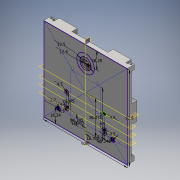
# Autodesk Inventor part: Complete Lifting Chassis with Balance and Variability
Saved by Autodesk Inventor 2016 (Build 200138000, 138)
## iProperties
Created: 2016-03-31
Part Number: Complete Lifting Chassis with Balance and Variability
Material: Generic
Document SubType Name: Modeling
Designer: Kenneth Daniel
Density: 1 g/cm^3
Appearance: Default
Author: Kenneth Daniel
## iProperties of the stored document Complete Lifting Chassis with Balance and Variability_3DPrint.ipt
Created: 2016-03-31
Part Number: Complete Lifting Chassis with Balance and Variability_3DPrint
Material: Generic
Document SubType Name: Modeling
Designer: Kenneth Daniel
Density: 1 g/cm^3
Appearance: Default
Author: Kenneth Daniel
Autodesk Inventor part; units mm, degrees
(part 1 of 2)
ref_plane "YZ Plane" through (0, 0, 0) normal (1, 0, 0) x (0, 1, 0)
ref_plane "XZ Plane" through (0, 0, 0) normal (0, 1, 0) x (-1, 0, 0)
sketch "Sketch1" plane through (0, 0, 0) normal (0, 1, 0) x (-1, 0, 0)
  line L0 (-46.4, 46.4) -> (-46.4, -46.4)
  line L1 (-46.4, -46.4) -> (46.4, -46.4)
  line L2 (46.4, -46.4) -> (46.4, 46.4)
  line L3 (46.4, 46.4) -> (-46.4, 46.4)
  line L4 (-46.4, 46.4) -> (46.4, -46.4) construction
  line L5 (-46.4, -46.4) -> (46.4, 46.4) construction
  line L6 (46.4, -46.4) -> (46.4, -30.16) construction
  line L7 (46.4, -30.16) -> (-46.4, -30.16) construction
  circle A0 centre (30.16, -30.16) radius 1.6
  circle A1 centre (30.16, -30.16) radius 2.2
  circle A2 centre (-30.16, -30.16) radius 1.6
  circle A3 centre (-30.16, -30.16) radius 2.2
  line L8 (0, 0) -> (0, -36.813) construction
  line L9 (0, -36.813) -> (16.702, -36.813) construction
  line L10 (0, -36.813) -> (-16.702, -36.813) construction
  line L11 (-16.702, -36.813) -> (-16.702, 14.187) construction
  line L12 (16.702, -36.813) -> (16.702, 14.187) construction
  line L13 (16.702, 14.187) -> (-16.702, 14.187) construction
  line L14 (16.702, -36.813) -> (16.702, -25.568) construction
  line L15 (16.702, -25.568) -> (21.202, -25.568) construction
  circle A4 centre (21.202, -25.568) radius 2.25
  line L16 (-16.702, -36.813) -> (-16.702, -25.568) construction
  line L17 (-16.702, -25.568) -> (-21.202, -25.568) construction
  line L18 (21.202, -25.568) -> (21.202, -9.693) construction
  circle A5 centre (21.202, -9.693) radius 2.25
  line L19 (-21.202, -25.568) -> (-21.202, -9.693) construction
  circle A6 centre (-21.202, -9.693) radius 2.25
  circle A7 centre (-21.202, -25.568) radius 2.25
  line L20 (0, 46.4) -> (0, 28.15) construction
  circle A8 centre (0, 28.15) radius 9.75
  circle A9 centre (0, 28.15) radius 6.2
  dimension "d0" = 92.8
  dimension "d1" = 92.8
  dimension "d2" = 16.24
  dimension "d3" = 3.2
  dimension "d4" = 4.4
  dimension "d5" = 3.2
  dimension "d6" = 4.4
  dimension "d7" = 36.813
  dimension "d8" = 16.702
  dimension "d9" = 16.702
  dimension "d10" = 51
  dimension "d11" = 11.245
  dimension "d12" = 4.5
  dimension "d13" = 4.5
  dimension "d15" = 4.5
  dimension "d16" = 11.245
  dimension "d18" = 15.875
  dimension "d19" = 4.5
  dimension "d22" = 4.5
  dimension "d23" = 4.5
  dimension "d24" = 18.25
  dimension "d25" = 19.5
  dimension "d26" = 12.4
  constraints: 42 end point, 10 centre point, 8 coincident, 8 point on line, 7 vertical, 5 perpendicular, 3 midpoint, 2 horizontal, 2 parallel
  measures "d0" distance of L0.start L0.end
  measures "d1" distance of L1.end L0.end
  measures "d2" distance of L1.end L6.end
  measures "d3" diameter of A0
  measures "d4" diameter of A1
  measures "d5" diameter of A2
  measures "d6" diameter of A3
  measures "d7" distance of L8.start L8.end
  measures "d8" distance of L8.end L9.end
  measures "d9" distance of L8.end L10.end
  measures "d10" distance of L10.end L11.end
  measures "d11" distance of L9.end L14.end
  measures "d12" distance of L14.end L15.end
  measures "d13" diameter of A4
  measures "d15" distance of L16.end L17.end
  measures "d16" distance of L10.end L16.end
  measures "d18" distance of L18.start L18.end
  measures "d19" diameter of A5
  measures "d22" diameter of A6
  measures "d23" diameter of A7
  measures "d24" distance of L20.start L20.end
  measures "d25" diameter of A8
  measures "d26" diameter of A9
extrude "Extrusion1" add sketch "Sketch1" along normal blind 5 contours L3 L2 L1 L0
extrude "Extrusion2" add sketch "Sketch1" along normal blind 1 contours A8
sketch "Sketch2" plane through (0, 1, 28.15) normal (0, 1, 0) x (1, 0, 0)
  circle A0 centre (0, 0) radius 9.75 projected
  circle A1 centre (0, 0) radius 6.2 projected
  circle A2 centre (0, 0) radius 6.2 projected
  circle A3 centre (0, 0) radius 9.75 projected
  line L0 (16.0737, 0.15) -> (6.1982, 0.15)
  line L1 (5.3373, 0.15) -> (5.3373, -0.15)
  line L2 (6.1982, -0.15) -> (16.0737, -0.15)
  line L3 (16.0737, -0.15) -> (16.0737, 0.15)
  line L4 (16.0737, 0.15) -> (5.3373, -0.15) construction
  line L5 (5.3373, 0.15) -> (16.0737, -0.15) construction
  circle A4 centre (0, 0) radius 6.2
  circle A5 centre (0, 0) radius 9.75
  circle A6 centre (0, 0) radius 6.2 projected
  line L6 (5.3373, 0.15) -> (9.7488, 0.15)
  line L7 (5.3373, -0.15) -> (9.7488, -0.15)
  arc A7 (4, -0.15) -> (3.9887, 0.15) centre (0, -0.15) ccw
  line L8 (5.3373, -0.15) -> (4, -0.15)
  line L9 (5.3373, 0.15) -> (3.9887, 0.15)
  point P0 (0, 28.15)
  point P1 (10.7055, 0)
  dimension "d35" = 0.3
  dimension "d43" = 8
  constraints: 20 end point, 8 point on circle, 3 centre point, 3 parallel, 3 point on line, 2 coincident, 2 midpoint, 1 horizontal, 1 perpendicular
  measures "d35" distance of L1.end L1.start
  measures "d43" diameter of A7
extrude "Extrusion5" add sketch "Sketch2" along normal up to surface (4 mm away) contours A0 L2 A1 L0 | A1 L7 L1 L6 | L1 L8 A7 L9 picked at (7.3832, -0.0333)
pattern_circular "Circular Pattern2" count 30 over 360 about axis through (0, 0, 28.15) along (0, 1, 0) of "Extrusion5"
sketch "Sketch4" plane through (0, 0, 0) normal (0, -1, 0) x (1, 0, 0)
  circle A0 centre (0, 28.15) radius 6.2 projected
  circle A1 centre (21.202, -25.568) radius 2.25 projected
  circle A2 centre (21.202, -9.693) radius 2.25 projected
  circle A3 centre (-21.202, -9.693) radius 2.25 projected
  circle A4 centre (-21.202, -25.568) radius 2.25 projected
  circle A5 centre (30.16, -30.16) radius 2.2 projected
  circle A6 centre (-30.16, -30.16) radius 2.2 projected
  line L0 (46.4, 46.4) -> (46.4, -46.4) projected
  line L1 (-46.4, 46.4) -> (46.4, 46.4) projected
  line L2 (-46.4, -46.4) -> (-46.4, 46.4) projected
  line L3 (46.4, -46.4) -> (-46.4, -46.4) projected
  circle A7 centre (0, 28.15) radius 3.9916
  circle A8 centre (0, 28.15) radius 4.3916
  point P0 (0, 0)
  dimension "d49" = 0.4
  constraints: 2 centre point, 1 coincident
  measures "d49" radial gap between concentric circles of A7 A8
extrude "Extrusion6" add sketch "Sketch4" against normal up to surface (1 mm away) contours A8
sketch "Sketch5" plane through (0, 5, 0) normal (0, 1, 0) x (1, 0, 0)
  circle A0 centre (0, -28.1477) radius 9.8088
  circle A1 centre (0, -28.1477) radius 6.2001
  point P0 (0, 0)
  constraints: 2 centre point, 1 coincident
extrude "Extrusion7" add sketch "Sketch5" against normal blind 0.5
sketch "Sketch6" plane through (0, 5, 0) normal (0, 1, 0) x (1, 0, 0)
  line L0 (46.4, -46.4) -> (46.4, 46.4) projected
  line L1 (46.4, 46.4) -> (-46.4, 46.4) projected
  line L2 (-46.4, 46.4) -> (-46.4, -46.4) projected
  line L3 (-46.4, -46.4) -> (46.4, -46.4) projected
  circle A0 centre (-30.16, 30.16) radius 2.2 projected
  circle A1 centre (30.16, 30.16) radius 2.2 projected
  circle A2 centre (-21.202, 25.568) radius 2.25 projected
  circle A3 centre (-21.202, 9.693) radius 2.25 projected
  circle A4 centre (21.202, 9.693) radius 2.25 projected
  circle A5 centre (21.202, 25.568) radius 2.25 projected
  line L4 (-3.9887, -28.3) -> (-6.1982, -28.3) projected
  arc A6 (-4, -28) -> (-3.9887, -28.3) centre (0, -28) ccw projected
  line L5 (-6.1983, -28) -> (-4, -28) projected
  arc A7 (-6.0944, -27.0079) -> (-6.1983, -28) centre (0, -28.1477) ccw projected
  line L6 (-3.9328, -27.4674) -> (-6.0944, -27.0079) projected
  arc A8 (-3.8814, -27.1716) -> (-3.9328, -27.4674) centre (0.0312, -28.0033) ccw projected
  line L7 (-6.0321, -26.7145) -> (-3.8814, -27.1716) projected
  arc A9 (-5.7242, -25.7656) -> (-6.0321, -26.7145) centre (0, -28.1477) ccw projected
  line L8 (-3.7049, -26.6647) -> (-5.7242, -25.7656) projected
  arc A10 (-3.5932, -26.386) -> (-3.7049, -26.6647) centre (0.061, -28.013) ccw projected
  line L9 (-5.6023, -25.4915) -> (-3.5932, -26.386) projected
  arc A11 (-5.1037, -24.6273) -> (-5.6023, -25.4915) centre (0, -28.1477) ccw projected
  line L10 (-3.3151, -25.9268) -> (-5.1037, -24.6273) projected
  arc A12 (-3.1479, -25.6775) -> (-3.3151, -25.9268) centre (0.0882, -28.0286) ccw projected
  line L11 (-4.9275, -24.3846) -> (-3.1479, -25.6775) projected
  arc A13 (-4.26, -23.6429) -> (-4.9275, -24.3846) centre (0, -28.1477) ccw projected
  line L12 (-2.7805, -25.2862) -> (-4.26, -23.6429) projected
  arc A14 (-2.5651, -25.0771) -> (-2.7805, -25.2862) centre (0.1115, -28.0496) ccw projected
  line L13 (-4.0371, -23.4421) -> (-2.5651, -25.0771) projected
  arc A15 (-3.23, -22.8555) -> (-4.0371, -23.4421) centre (0, -28.1477) ccw projected
  line L14 (-2.1243, -24.7707) -> (-3.23, -22.8555) projected
  arc A16 (-1.8701, -24.6109) -> (-2.1243, -24.7707) centre (0.1299, -28.075) ccw projected
  line L15 (-2.9702, -22.7054) -> (-1.8701, -24.6109) projected
  arc A17 (-2.0587, -22.2994) -> (-2.9702, -22.7054) centre (0, -28.1477) ccw projected
  line L16 (-1.3752, -24.4028) -> (-2.0587, -22.2994) projected
  arc A18 (-1.0934, -24.2994) -> (-1.3752, -24.4028) centre (0.1427, -28.1036) ccw projected
  line L17 (-1.7734, -22.2067) -> (-1.0934, -24.2994) projected
  arc A19 (-0.7973, -21.9991) -> (-1.7734, -22.2067) centre (0, -28.1477) ccw projected
  line L18 (-0.5661, -24.1988) -> (-0.7973, -21.9991) projected
  arc A20 (-0.2689, -24.1562) -> (-0.5661, -24.1988) centre (0.1492, -28.1343) ccw projected
  line L19 (-0.499, -21.9677) -> (-0.2689, -24.1562) projected
  arc A21 (0.499, -21.9677) -> (-0.499, -21.9677) centre (0, -28.1477) ccw projected
  line L20 (0.2678, -24.1674) -> (0.499, -21.9677) projected
  arc A22 (0.5673, -24.1876) -> (0.2678, -24.1674) centre (0.1492, -28.1657) ccw projected
  line L21 (0.7973, -21.9991) -> (0.5673, -24.1876) projected
  arc A23 (1.7734, -22.2067) -> (0.7973, -21.9991) centre (0, -28.1477) ccw projected
  line L22 (1.0899, -24.3101) -> (1.7734, -22.2067) projected
  arc A24 (1.3787, -24.3921) -> (1.0899, -24.3101) centre (0.1427, -28.1964) ccw projected
  line L23 (2.0587, -22.2994) -> (1.3787, -24.3921) projected
  arc A25 (2.9702, -22.7054) -> (2.0587, -22.2994) centre (0, -28.1477) ccw projected
  line L24 (1.8645, -24.6207) -> (2.9702, -22.7054) projected
  arc A26 (2.1299, -24.7609) -> (1.8645, -24.6207) centre (0.1299, -28.225) ccw projected
  line L25 (3.23, -22.8555) -> (2.1299, -24.7609) projected
  arc A27 (4.0371, -23.4421) -> (3.23, -22.8555) centre (0, -28.1477) ccw projected
  line L26 (2.5575, -25.0854) -> (4.0371, -23.4421) projected
  arc A28 (2.788, -25.2778) -> (2.5575, -25.0854) centre (0.1115, -28.2504) ccw projected
  line L27 (4.26, -23.6429) -> (2.788, -25.2778) projected
  arc A29 (4.9275, -24.3846) -> (4.26, -23.6429) centre (0, -28.1477) ccw projected
  line L28 (3.1388, -25.6841) -> (4.9275, -24.3846) projected
  arc A30 (3.3242, -25.9202) -> (3.1388, -25.6841) centre (0.0882, -28.2714) ccw projected
  line L29 (5.1037, -24.6273) -> (3.3242, -25.9202) projected
  arc A31 (5.6023, -25.4915) -> (5.1037, -24.6273) centre (0, -28.1477) ccw projected
  line L30 (3.5829, -26.3906) -> (5.6023, -25.4915) projected
  arc A32 (3.7152, -26.6601) -> (3.5829, -26.3906) centre (0.061, -28.287) ccw projected
  line L31 (5.7242, -25.7656) -> (3.7152, -26.6601) projected
  arc A33 (6.0321, -26.7145) -> (5.7242, -25.7656) centre (0, -28.1477) ccw projected
  line L32 (3.8704, -27.174) -> (6.0321, -26.7145) projected
  arc A34 (3.9438, -27.4651) -> (3.8704, -27.174) centre (0.0312, -28.2967) ccw projected
  line L33 (6.0944, -27.0079) -> (3.9438, -27.4651) projected
  arc A35 (6.1983, -28) -> (6.0944, -27.0079) centre (0, -28.1477) ccw projected
  line L34 (3.9887, -28) -> (6.1983, -28) projected
  arc A36 (4, -28.3) -> (3.9887, -28) centre (0, -28.3) ccw projected
  line L35 (6.1982, -28.3) -> (4, -28.3) projected
  arc A37 (6.0936, -29.2919) -> (6.1982, -28.3) centre (0, -28.1477) ccw projected
  line L36 (3.9328, -28.8326) -> (6.0936, -29.2919) projected
  arc A38 (3.8814, -29.1284) -> (3.9328, -28.8326) centre (-0.0312, -28.2967) ccw projected
  line L37 (6.0311, -29.5853) -> (3.8814, -29.1284) projected
  arc A39 (5.7226, -30.5337) -> (6.0311, -29.5853) centre (0, -28.1477) ccw projected
  line L38 (3.7049, -29.6353) -> (5.7226, -30.5337) projected
  arc A40 (3.5932, -29.914) -> (3.7049, -29.6353) centre (-0.061, -28.287) ccw projected
  line L39 (5.6005, -30.8077) -> (3.5932, -29.914) projected
  arc A41 (5.1016, -31.6711) -> (5.6005, -30.8077) centre (0, -28.1477) ccw projected
  line L40 (3.3151, -30.3732) -> (5.1016, -31.6711) projected
  arc A42 (3.1479, -30.6225) -> (3.3151, -30.3732) centre (-0.0882, -28.2714) ccw projected
  line L41 (4.9252, -31.9138) -> (3.1479, -30.6225) projected
  arc A43 (4.2578, -32.6546) -> (4.9252, -31.9138) centre (0, -28.1477) ccw projected
  line L42 (2.7805, -31.0138) -> (4.2578, -32.6546) projected
  arc A44 (2.5651, -31.2229) -> (2.7805, -31.0138) centre (-0.1115, -28.2504) ccw projected
  line L43 (4.0348, -32.8553) -> (2.5651, -31.2229) projected
  arc A45 (3.228, -33.4411) -> (4.0348, -32.8553) centre (0, -28.1477) ccw projected
  line L44 (2.1243, -31.5293) -> (3.228, -33.4411) projected
  arc A46 (1.8701, -31.6891) -> (2.1243, -31.5293) centre (-0.1299, -28.225) ccw projected
  line L45 (2.9682, -33.5911) -> (1.8701, -31.6891) projected
  arc A47 (2.0573, -33.9964) -> (2.9682, -33.5911) centre (0, -28.1477) ccw projected
  line L46 (1.3752, -31.8972) -> (2.0573, -33.9964) projected
  arc A48 (1.0934, -32.0006) -> (1.3752, -31.8972) centre (-0.1427, -28.1964) ccw projected
  line L47 (1.772, -34.0891) -> (1.0934, -32.0006) projected
  arc A49 (0.7968, -34.2963) -> (1.772, -34.0891) centre (0, -28.1477) ccw projected
  line L48 (0.5661, -32.1012) -> (0.7968, -34.2963) projected
  arc A50 (0.2689, -32.1438) -> (0.5661, -32.1012) centre (-0.1492, -28.1657) ccw projected
  line L49 (0.4985, -34.3277) -> (0.2689, -32.1438) projected
  arc A51 (-0.4985, -34.3277) -> (0.4985, -34.3277) centre (0, -28.1477) ccw projected
  line L50 (-0.2678, -32.1326) -> (-0.4985, -34.3277) projected
  arc A52 (-0.5673, -32.1124) -> (-0.2678, -32.1326) centre (-0.1492, -28.1343) ccw projected
  line L51 (-0.7968, -34.2963) -> (-0.5673, -32.1124) projected
  arc A53 (-1.772, -34.0891) -> (-0.7968, -34.2963) centre (0, -28.1477) ccw projected
  line L52 (-1.0899, -31.9899) -> (-1.772, -34.0891) projected
  arc A54 (-1.3787, -31.9079) -> (-1.0899, -31.9899) centre (-0.1427, -28.1036) ccw projected
  line L53 (-2.0573, -33.9964) -> (-1.3787, -31.9079) projected
  arc A55 (-2.9682, -33.5911) -> (-2.0573, -33.9964) centre (0, -28.1477) ccw projected
  line L54 (-1.8645, -31.6793) -> (-2.9682, -33.5911) projected
  arc A56 (-2.1299, -31.5391) -> (-1.8645, -31.6793) centre (-0.1299, -28.075) ccw projected
  line L55 (-3.228, -33.4411) -> (-2.1299, -31.5391) projected
  arc A57 (-4.0348, -32.8553) -> (-3.228, -33.4411) centre (0, -28.1477) ccw projected
  line L56 (-2.5575, -31.2146) -> (-4.0348, -32.8553) projected
  arc A58 (-2.788, -31.0222) -> (-2.5575, -31.2146) centre (-0.1115, -28.0496) ccw projected
  line L57 (-4.2578, -32.6546) -> (-2.788, -31.0222) projected
  arc A59 (-4.9252, -31.9138) -> (-4.2578, -32.6546) centre (0, -28.1477) ccw projected
  line L58 (-3.1388, -30.6159) -> (-4.9252, -31.9138) projected
  arc A60 (-3.3242, -30.3798) -> (-3.1388, -30.6159) centre (-0.0882, -28.0286) ccw projected
  line L59 (-5.1016, -31.6711) -> (-3.3242, -30.3798) projected
  arc A61 (-5.6005, -30.8077) -> (-5.1016, -31.6711) centre (0, -28.1477) ccw projected
  line L60 (-3.5829, -29.9094) -> (-5.6005, -30.8077) projected
  arc A62 (-3.7152, -29.6399) -> (-3.5829, -29.9094) centre (-0.061, -28.013) ccw projected
  line L61 (-5.7226, -30.5337) -> (-3.7152, -29.6399) projected
  arc A63 (-6.0311, -29.5853) -> (-5.7226, -30.5337) centre (0, -28.1477) ccw projected
  line L62 (-3.8704, -29.126) -> (-6.0311, -29.5853) projected
  arc A64 (-3.9438, -28.8349) -> (-3.8704, -29.126) centre (-0.0312, -28.0033) ccw projected
  line L63 (-6.0936, -29.2919) -> (-3.9438, -28.8349) projected
  arc A65 (-6.1982, -28.3) -> (-6.0936, -29.2919) centre (0, -28.1477) ccw projected
  circle A66 centre (-21.202, 9.693) radius 2.25 projected
  line L64 (-19.3895, 11.0261) -> (-23.0065, 8.349) construction
  line L65 (-19.332, 10.9442) -> (-20.3393, 10.1987)
  line L66 (-21.9377, 9.0157) -> (-22.945, 8.2701)
  line L67 (-19.4505, 11.1054) -> (-20.4572, 10.3603)
  line L68 (-22.0578, 9.1756) -> (-23.0644, 8.4305)
  arc A67 (-22.0578, 9.1756) -> (-21.9377, 9.0157) centre (-21.202, 9.693) ccw
  arc A68 (-20.3393, 10.1987) -> (-20.4572, 10.3603) centre (-21.202, 9.693) ccw
  point P0 (0, 0)
  constraints: 16 point on circle, 10 end point, 2 centre point, 2 parallel, 1 coincident, 1 other
extrude "Extrusion8" add sketch "Sketch6" against normal up to surface (5 mm away) contours L65 A68 L67 A3 | A3 L68 A67 L66
pattern_circular "Circular Pattern3" count 10 over 360 about axis through (-21.202, 0, -9.693) along (0, 1, 0) of "Extrusion8"
ref_plane "Work Plane3" through (-21.202, 0, -9.693) normal (0, 0, 1) x (1, 0, 0)
ref_plane "Work Plane5" through (-21.202, 0, -17.6305) normal (0, 0, 1) x (1, 0, 0)
ref_plane "Work Plane4" through (-21.202, 0, -25.568) normal (0, 0, 1) x (1, 0, 0)
mirror "Mirror1" about plane through (-21.202, 0, -17.6305) normal (0, 0, 1) of "Extrusion8", "Circular Pattern3"
ref_plane "Work Plane6" through (0, 0, -46.4) normal (-1, 0, 0) x (0, 0, 1)
mirror "Mirror2" about plane through (0, 0, -46.4) normal (-1, 0, 0) of "Extrusion8", "Circular Pattern3", "Mirror1"
sketch "Sketch7" plane through (0, 5, 0) normal (0, 1, 0) x (1, 0, 0)
  arc A0 (20.3393, 25.0623) -> (20.4663, 24.8907) centre (21.202, 25.568) ccw projected
  line L0 (20.3393, 25.0623) -> (19.332, 24.3168) projected
  arc A1 (18.9556, 25.4414) -> (19.332, 24.3168) centre (21.202, 25.568) ccw projected
  line L1 (18.9556, 25.4414) -> (20.2087, 25.4525) projected
  arc A2 (20.2068, 25.666) -> (20.2087, 25.4525) centre (21.202, 25.568) ccw projected
  line L2 (20.2068, 25.666) -> (18.9537, 25.6549) projected
  arc A3 (19.3102, 26.786) -> (18.9537, 25.6549) centre (21.202, 25.568) ccw projected
  line L3 (19.3102, 26.786) -> (20.3305, 26.0584) projected
  arc A4 (20.4545, 26.2322) -> (20.3305, 26.0584) centre (21.202, 25.568) ccw projected
  line L4 (20.4545, 26.2322) -> (19.4341, 26.9598) projected
  arc A5 (20.3874, 27.6654) -> (19.4341, 26.9598) centre (21.202, 25.568) ccw projected
  line L5 (20.3874, 27.6654) -> (20.7852, 26.477) projected
  arc A6 (20.9876, 26.5448) -> (20.7852, 26.477) centre (21.202, 25.568) ccw projected
  line L6 (20.9876, 26.5448) -> (20.5899, 27.7331) projected
  arc A7 (21.7758, 27.7436) -> (20.5899, 27.7331) centre (21.202, 25.568) ccw projected
  line L7 (21.7758, 27.7436) -> (21.3991, 26.5484) projected
  arc A8 (21.6027, 26.4842) -> (21.3991, 26.5484) centre (21.202, 25.568) ccw projected
  line L8 (21.6027, 26.4842) -> (21.9794, 27.6794) projected
  arc A9 (22.945, 26.9909) -> (21.9794, 27.6794) centre (21.202, 25.568) ccw projected
  line L9 (22.945, 26.9909) -> (21.9377, 26.2453) projected
  arc A10 (22.0647, 26.0737) -> (21.9377, 26.2453) centre (21.202, 25.568) ccw projected
  line L10 (22.0647, 26.0737) -> (23.072, 26.8192) projected
  arc A11 (23.4484, 25.6946) -> (23.072, 26.8192) centre (21.202, 25.568) ccw projected
  line L11 (23.4484, 25.6946) -> (22.1953, 25.6835) projected
  arc A12 (22.1972, 25.47) -> (22.1953, 25.6835) centre (21.202, 25.568) ccw projected
  line L12 (22.1972, 25.47) -> (23.4503, 25.4811) projected
  arc A13 (23.0938, 24.35) -> (23.4503, 25.4811) centre (21.202, 25.568) ccw projected
  line L13 (23.0938, 24.35) -> (22.0735, 25.0776) projected
  arc A14 (21.9495, 24.9038) -> (22.0735, 25.0776) centre (21.202, 25.568) ccw projected
  line L14 (21.9495, 24.9038) -> (22.9699, 24.1762) projected
  arc A15 (22.0166, 23.4706) -> (22.9699, 24.1762) centre (21.202, 25.568) ccw projected
  line L15 (22.0166, 23.4706) -> (21.6188, 24.659) projected
  arc A16 (21.4164, 24.5912) -> (21.6188, 24.659) centre (21.202, 25.568) ccw projected
  line L16 (21.4164, 24.5912) -> (21.8141, 23.4029) projected
  arc A17 (20.6282, 23.3924) -> (21.8141, 23.4029) centre (21.202, 25.568) ccw projected
  line L17 (20.6282, 23.3924) -> (21.0049, 24.5876) projected
  arc A18 (20.8013, 24.6518) -> (21.0049, 24.5876) centre (21.202, 25.568) ccw projected
  line L18 (20.8013, 24.6518) -> (20.4246, 23.4566) projected
  arc A19 (19.459, 24.1451) -> (20.4246, 23.4566) centre (21.202, 25.568) ccw projected
  line L19 (19.459, 24.1451) -> (20.4663, 24.8907) projected
  arc A20 (-20.4663, 24.8907) -> (-20.3393, 25.0623) centre (-21.202, 25.568) ccw projected
  line L20 (-19.459, 24.1451) -> (-20.4663, 24.8907) projected
  arc A21 (-20.4246, 23.4566) -> (-19.459, 24.1451) centre (-21.202, 25.568) ccw projected
  line L21 (-20.8013, 24.6518) -> (-20.4246, 23.4566) projected
  arc A22 (-21.0049, 24.5876) -> (-20.8013, 24.6518) centre (-21.202, 25.568) ccw projected
  line L22 (-20.6282, 23.3924) -> (-21.0049, 24.5876) projected
  arc A23 (-21.8141, 23.4029) -> (-20.6282, 23.3924) centre (-21.202, 25.568) ccw projected
  line L23 (-21.4164, 24.5912) -> (-21.8141, 23.4029) projected
  arc A24 (-21.6188, 24.659) -> (-21.4164, 24.5912) centre (-21.202, 25.568) ccw projected
  line L24 (-22.0166, 23.4706) -> (-21.6188, 24.659) projected
  arc A25 (-22.9699, 24.1762) -> (-22.0166, 23.4706) centre (-21.202, 25.568) ccw projected
  line L25 (-21.9495, 24.9038) -> (-22.9699, 24.1762) projected
  arc A26 (-22.0735, 25.0776) -> (-21.9495, 24.9038) centre (-21.202, 25.568) ccw projected
  line L26 (-23.0938, 24.35) -> (-22.0735, 25.0776) projected
  arc A27 (-23.4503, 25.4811) -> (-23.0938, 24.35) centre (-21.202, 25.568) ccw projected
  line L27 (-22.1972, 25.47) -> (-23.4503, 25.4811) projected
  arc A28 (-22.1953, 25.6835) -> (-22.1972, 25.47) centre (-21.202, 25.568) ccw projected
  line L28 (-23.4484, 25.6946) -> (-22.1953, 25.6835) projected
  arc A29 (-23.072, 26.8192) -> (-23.4484, 25.6946) centre (-21.202, 25.568) ccw projected
  line L29 (-22.0647, 26.0737) -> (-23.072, 26.8192) projected
  arc A30 (-21.9377, 26.2453) -> (-22.0647, 26.0737) centre (-21.202, 25.568) ccw projected
  line L30 (-22.945, 26.9909) -> (-21.9377, 26.2453) projected
  arc A31 (-21.9794, 27.6794) -> (-22.945, 26.9909) centre (-21.202, 25.568) ccw projected
  line L31 (-21.6027, 26.4842) -> (-21.9794, 27.6794) projected
  arc A32 (-21.3991, 26.5484) -> (-21.6027, 26.4842) centre (-21.202, 25.568) ccw projected
  line L32 (-21.7758, 27.7436) -> (-21.3991, 26.5484) projected
  arc A33 (-20.5899, 27.7331) -> (-21.7758, 27.7436) centre (-21.202, 25.568) ccw projected
  line L33 (-20.9876, 26.5448) -> (-20.5899, 27.7331) projected
  arc A34 (-20.7852, 26.477) -> (-20.9876, 26.5448) centre (-21.202, 25.568) ccw projected
  line L34 (-20.3874, 27.6654) -> (-20.7852, 26.477) projected
  arc A35 (-19.4341, 26.9598) -> (-20.3874, 27.6654) centre (-21.202, 25.568) ccw projected
  line L35 (-20.4545, 26.2322) -> (-19.4341, 26.9598) projected
  arc A36 (-20.3305, 26.0584) -> (-20.4545, 26.2322) centre (-21.202, 25.568) ccw projected
  line L36 (-19.3102, 26.786) -> (-20.3305, 26.0584) projected
  arc A37 (-18.9537, 25.6549) -> (-19.3102, 26.786) centre (-21.202, 25.568) ccw projected
  line L37 (-20.2068, 25.666) -> (-18.9537, 25.6549) projected
  arc A38 (-20.2087, 25.4525) -> (-20.2068, 25.666) centre (-21.202, 25.568) ccw projected
  line L38 (-18.9556, 25.4414) -> (-20.2087, 25.4525) projected
  arc A39 (-19.332, 24.3168) -> (-18.9556, 25.4414) centre (-21.202, 25.568) ccw projected
  line L39 (-20.3393, 25.0623) -> (-19.332, 24.3168) projected
  arc A40 (-20.3393, 10.1987) -> (-20.4663, 10.3703) centre (-21.202, 9.693) ccw projected
  line L40 (-20.3393, 10.1987) -> (-19.332, 10.9442) projected
  arc A41 (-18.9556, 9.8196) -> (-19.332, 10.9442) centre (-21.202, 9.693) ccw projected
  line L41 (-18.9556, 9.8196) -> (-20.2087, 9.8085) projected
  arc A42 (-20.2068, 9.595) -> (-20.2087, 9.8085) centre (-21.202, 9.693) ccw projected
  line L42 (-20.2068, 9.595) -> (-18.9537, 9.6061) projected
  arc A43 (-19.3102, 8.475) -> (-18.9537, 9.6061) centre (-21.202, 9.693) ccw projected
  line L43 (-19.3102, 8.475) -> (-20.3305, 9.2026) projected
  arc A44 (-20.4545, 9.0288) -> (-20.3305, 9.2026) centre (-21.202, 9.693) ccw projected
  line L44 (-20.4545, 9.0288) -> (-19.4341, 8.3012) projected
  arc A45 (-20.3874, 7.5956) -> (-19.4341, 8.3012) centre (-21.202, 9.693) ccw projected
  line L45 (-20.3874, 7.5956) -> (-20.7852, 8.784) projected
  arc A46 (-20.9876, 8.7162) -> (-20.7852, 8.784) centre (-21.202, 9.693) ccw projected
  line L46 (-20.9876, 8.7162) -> (-20.5899, 7.5279) projected
  arc A47 (-21.7758, 7.5174) -> (-20.5899, 7.5279) centre (-21.202, 9.693) ccw projected
  line L47 (-21.7758, 7.5174) -> (-21.3991, 8.7126) projected
  arc A48 (-21.6027, 8.7768) -> (-21.3991, 8.7126) centre (-21.202, 9.693) ccw projected
  line L48 (-21.6027, 8.7768) -> (-21.9794, 7.5816) projected
  arc A49 (-22.945, 8.2701) -> (-21.9794, 7.5816) centre (-21.202, 9.693) ccw projected
  line L49 (-22.945, 8.2701) -> (-21.9377, 9.0157) projected
  arc A50 (-22.0647, 9.1873) -> (-21.9377, 9.0157) centre (-21.202, 9.693) ccw projected
  line L50 (-22.0647, 9.1873) -> (-23.072, 8.4418) projected
  arc A51 (-23.4484, 9.5664) -> (-23.072, 8.4418) centre (-21.202, 9.693) ccw projected
  line L51 (-23.4484, 9.5664) -> (-22.1953, 9.5775) projected
  arc A52 (-22.1972, 9.791) -> (-22.1953, 9.5775) centre (-21.202, 9.693) ccw projected
  line L52 (-22.1972, 9.791) -> (-23.4503, 9.7799) projected
  arc A53 (-23.0938, 10.911) -> (-23.4503, 9.7799) centre (-21.202, 9.693) ccw projected
  line L53 (-23.0938, 10.911) -> (-22.0735, 10.1834) projected
  arc A54 (-21.9495, 10.3572) -> (-22.0735, 10.1834) centre (-21.202, 9.693) ccw projected
  line L54 (-21.9495, 10.3572) -> (-22.9699, 11.0848) projected
  arc A55 (-22.0166, 11.7904) -> (-22.9699, 11.0848) centre (-21.202, 9.693) ccw projected
  line L55 (-22.0166, 11.7904) -> (-21.6188, 10.602) projected
  arc A56 (-21.4164, 10.6698) -> (-21.6188, 10.602) centre (-21.202, 9.693) ccw projected
  line L56 (-21.4164, 10.6698) -> (-21.8141, 11.8581) projected
  arc A57 (-20.6282, 11.8686) -> (-21.8141, 11.8581) centre (-21.202, 9.693) ccw projected
  line L57 (-20.6282, 11.8686) -> (-21.0049, 10.6734) projected
  arc A58 (-20.8013, 10.6092) -> (-21.0049, 10.6734) centre (-21.202, 9.693) ccw projected
  line L58 (-20.8013, 10.6092) -> (-20.4246, 11.8044) projected
  arc A59 (-19.459, 11.1159) -> (-20.4246, 11.8044) centre (-21.202, 9.693) ccw projected
  line L59 (-19.459, 11.1159) -> (-20.4663, 10.3703) projected
  line L60 (46.4, -46.4) -> (46.4, 46.4) projected
  line L61 (46.4, 46.4) -> (-46.4, 46.4) projected
  line L62 (-46.4, 46.4) -> (-46.4, -46.4) projected
  line L63 (-46.4, -46.4) -> (46.4, -46.4) projected
  circle A60 centre (-30.16, 30.16) radius 2.2 projected
  circle A61 centre (30.16, 30.16) radius 2.2 projected
  line L64 (-3.9887, -28.3) -> (-6.1982, -28.3) projected
  arc A62 (-4, -28) -> (-3.9887, -28.3) centre (0, -28) ccw projected
  line L65 (-6.1983, -28) -> (-4, -28) projected
  arc A63 (-6.0944, -27.0079) -> (-6.1983, -28) centre (0, -28.1477) ccw projected
  line L66 (-3.9328, -27.4674) -> (-6.0944, -27.0079) projected
  arc A64 (-3.8814, -27.1716) -> (-3.9328, -27.4674) centre (0.0312, -28.0033) ccw projected
  line L67 (-6.0321, -26.7145) -> (-3.8814, -27.1716) projected
  arc A65 (-5.7242, -25.7656) -> (-6.0321, -26.7145) centre (0, -28.1477) ccw projected
  line L68 (-3.7049, -26.6647) -> (-5.7242, -25.7656) projected
  arc A66 (-3.5932, -26.386) -> (-3.7049, -26.6647) centre (0.061, -28.013) ccw projected
  line L69 (-5.6023, -25.4915) -> (-3.5932, -26.386) projected
  arc A67 (-5.1037, -24.6273) -> (-5.6023, -25.4915) centre (0, -28.1477) ccw projected
  line L70 (-3.3151, -25.9268) -> (-5.1037, -24.6273) projected
  arc A68 (-3.1479, -25.6775) -> (-3.3151, -25.9268) centre (0.0882, -28.0286) ccw projected
  line L71 (-4.9275, -24.3846) -> (-3.1479, -25.6775) projected
  arc A69 (-4.26, -23.6429) -> (-4.9275, -24.3846) centre (0, -28.1477) ccw projected
  line L72 (-2.7805, -25.2862) -> (-4.26, -23.6429) projected
  arc A70 (-2.5651, -25.0771) -> (-2.7805, -25.2862) centre (0.1115, -28.0496) ccw projected
  line L73 (-4.0371, -23.4421) -> (-2.5651, -25.0771) projected
  arc A71 (-3.23, -22.8555) -> (-4.0371, -23.4421) centre (0, -28.1477) ccw projected
  line L74 (-2.1243, -24.7707) -> (-3.23, -22.8555) projected
  arc A72 (-1.8701, -24.6109) -> (-2.1243, -24.7707) centre (0.1299, -28.075) ccw projected
  line L75 (-2.9702, -22.7054) -> (-1.8701, -24.6109) projected
  arc A73 (-2.0587, -22.2994) -> (-2.9702, -22.7054) centre (0, -28.1477) ccw projected
  line L76 (-1.3752, -24.4028) -> (-2.0587, -22.2994) projected
  arc A74 (-1.0934, -24.2994) -> (-1.3752, -24.4028) centre (0.1427, -28.1036) ccw projected
  line L77 (-1.7734, -22.2067) -> (-1.0934, -24.2994) projected
  arc A75 (-0.7973, -21.9991) -> (-1.7734, -22.2067) centre (0, -28.1477) ccw projected
  line L78 (-0.5661, -24.1988) -> (-0.7973, -21.9991) projected
  arc A76 (-0.2689, -24.1562) -> (-0.5661, -24.1988) centre (0.1492, -28.1343) ccw projected
  line L79 (-0.499, -21.9677) -> (-0.2689, -24.1562) projected
  arc A77 (0.499, -21.9677) -> (-0.499, -21.9677) centre (0, -28.1477) ccw projected
  line L80 (0.2678, -24.1674) -> (0.499, -21.9677) projected
  arc A78 (0.5673, -24.1876) -> (0.2678, -24.1674) centre (0.1492, -28.1657) ccw projected
  line L81 (0.7973, -21.9991) -> (0.5673, -24.1876) projected
  arc A79 (1.7734, -22.2067) -> (0.7973, -21.9991) centre (0, -28.1477) ccw projected
  line L82 (1.0899, -24.3101) -> (1.7734, -22.2067) projected
  arc A80 (1.3787, -24.3921) -> (1.0899, -24.3101) centre (0.1427, -28.1964) ccw projected
  line L83 (2.0587, -22.2994) -> (1.3787, -24.3921) projected
  arc A81 (2.9702, -22.7054) -> (2.0587, -22.2994) centre (0, -28.1477) ccw projected
  line L84 (1.8645, -24.6207) -> (2.9702, -22.7054) projected
  arc A82 (2.1299, -24.7609) -> (1.8645, -24.6207) centre (0.1299, -28.225) ccw projected
  line L85 (3.23, -22.8555) -> (2.1299, -24.7609) projected
  arc A83 (4.0371, -23.4421) -> (3.23, -22.8555) centre (0, -28.1477) ccw projected
  line L86 (2.5575, -25.0854) -> (4.0371, -23.4421) projected
  arc A84 (2.788, -25.2778) -> (2.5575, -25.0854) centre (0.1115, -28.2504) ccw projected
  line L87 (4.26, -23.6429) -> (2.788, -25.2778) projected
  arc A85 (4.9275, -24.3846) -> (4.26, -23.6429) centre (0, -28.1477) ccw projected
  line L88 (3.1388, -25.6841) -> (4.9275, -24.3846) projected
  arc A86 (3.3242, -25.9202) -> (3.1388, -25.6841) centre (0.0882, -28.2714) ccw projected
  line L89 (5.1037, -24.6273) -> (3.3242, -25.9202) projected
  arc A87 (5.6023, -25.4915) -> (5.1037, -24.6273) centre (0, -28.1477) ccw projected
  line L90 (3.5829, -26.3906) -> (5.6023, -25.4915) projected
  arc A88 (3.7152, -26.6601) -> (3.5829, -26.3906) centre (0.061, -28.287) ccw projected
  line L91 (5.7242, -25.7656) -> (3.7152, -26.6601) projected
  arc A89 (6.0321, -26.7145) -> (5.7242, -25.7656) centre (0, -28.1477) ccw projected
  line L92 (3.8704, -27.174) -> (6.0321, -26.7145) projected
  arc A90 (3.9438, -27.4651) -> (3.8704, -27.174) centre (0.0312, -28.2967) ccw projected
  line L93 (6.0944, -27.0079) -> (3.9438, -27.4651) projected
  arc A91 (6.1983, -28) -> (6.0944, -27.0079) centre (0, -28.1477) ccw projected
  line L94 (3.9887, -28) -> (6.1983, -28) projected
  arc A92 (4, -28.3) -> (3.9887, -28) centre (0, -28.3) ccw projected
  line L95 (6.1982, -28.3) -> (4, -28.3) projected
  arc A93 (6.0936, -29.2919) -> (6.1982, -28.3) centre (0, -28.1477) ccw projected
  line L96 (3.9328, -28.8326) -> (6.0936, -29.2919) projected
  arc A94 (3.8814, -29.1284) -> (3.9328, -28.8326) centre (-0.0312, -28.2967) ccw projected
  line L97 (6.0311, -29.5853) -> (3.8814, -29.1284) projected
  arc A95 (5.7226, -30.5337) -> (6.0311, -29.5853) centre (0, -28.1477) ccw projected
  line L98 (3.7049, -29.6353) -> (5.7226, -30.5337) projected
  arc A96 (3.5932, -29.914) -> (3.7049, -29.6353) centre (-0.061, -28.287) ccw projected
  line L99 (5.6005, -30.8077) -> (3.5932, -29.914) projected
  arc A97 (5.1016, -31.6711) -> (5.6005, -30.8077) centre (0, -28.1477) ccw projected
  line L100 (3.3151, -30.3732) -> (5.1016, -31.6711) projected
  arc A98 (3.1479, -30.6225) -> (3.3151, -30.3732) centre (-0.0882, -28.2714) ccw projected
  line L101 (4.9252, -31.9138) -> (3.1479, -30.6225) projected
  arc A99 (4.2578, -32.6546) -> (4.9252, -31.9138) centre (0, -28.1477) ccw projected
  line L102 (2.7805, -31.0138) -> (4.2578, -32.6546) projected
  arc A100 (2.5651, -31.2229) -> (2.7805, -31.0138) centre (-0.1115, -28.2504) ccw projected
  line L103 (4.0348, -32.8553) -> (2.5651, -31.2229) projected
  arc A101 (3.228, -33.4411) -> (4.0348, -32.8553) centre (0, -28.1477) ccw projected
  line L104 (2.1243, -31.5293) -> (3.228, -33.4411) projected
  arc A102 (1.8701, -31.6891) -> (2.1243, -31.5293) centre (-0.1299, -28.225) ccw projected
  line L105 (2.9682, -33.5911) -> (1.8701, -31.6891) projected
  arc A103 (2.0573, -33.9964) -> (2.9682, -33.5911) centre (0, -28.1477) ccw projected
  line L106 (1.3752, -31.8972) -> (2.0573, -33.9964) projected
  arc A104 (1.0934, -32.0006) -> (1.3752, -31.8972) centre (-0.1427, -28.1964) ccw projected
  line L107 (1.772, -34.0891) -> (1.0934, -32.0006) projected
  arc A105 (0.7968, -34.2963) -> (1.772, -34.0891) centre (0, -28.1477) ccw projected
  line L108 (0.5661, -32.1012) -> (0.7968, -34.2963) projected
  arc A106 (0.2689, -32.1438) -> (0.5661, -32.1012) centre (-0.1492, -28.1657) ccw projected
  line L109 (0.4985, -34.3277) -> (0.2689, -32.1438) projected
  arc A107 (-0.4985, -34.3277) -> (0.4985, -34.3277) centre (0, -28.1477) ccw projected
  line L110 (-0.2678, -32.1326) -> (-0.4985, -34.3277) projected
  arc A108 (-0.5673, -32.1124) -> (-0.2678, -32.1326) centre (-0.1492, -28.1343) ccw projected
  line L111 (-0.7968, -34.2963) -> (-0.5673, -32.1124) projected
  arc A109 (-1.772, -34.0891) -> (-0.7968, -34.2963) centre (0, -28.1477) ccw projected
  line L112 (-1.0899, -31.9899) -> (-1.772, -34.0891) projected
  arc A110 (-1.3787, -31.9079) -> (-1.0899, -31.9899) centre (-0.1427, -28.1036) ccw projected
  line L113 (-2.0573, -33.9964) -> (-1.3787, -31.9079) projected
  arc A111 (-2.9682, -33.5911) -> (-2.0573, -33.9964) centre (0, -28.1477) ccw projected
  line L114 (-1.8645, -31.6793) -> (-2.9682, -33.5911) projected
  arc A112 (-2.1299, -31.5391) -> (-1.8645, -31.6793) centre (-0.1299, -28.075) ccw projected
  line L115 (-3.228, -33.4411) -> (-2.1299, -31.5391) projected
  arc A113 (-4.0348, -32.8553) -> (-3.228, -33.4411) centre (0, -28.1477) ccw projected
  line L116 (-2.5575, -31.2146) -> (-4.0348, -32.8553) projected
  arc A114 (-2.788, -31.0222) -> (-2.5575, -31.2146) centre (-0.1115, -28.0496) ccw projected
  line L117 (-4.2578, -32.6546) -> (-2.788, -31.0222) projected
  arc A115 (-4.9252, -31.9138) -> (-4.2578, -32.6546) centre (0, -28.1477) ccw projected
  line L118 (-3.1388, -30.6159) -> (-4.9252, -31.9138) projected
  arc A116 (-3.3242, -30.3798) -> (-3.1388, -30.6159) centre (-0.0882, -28.0286) ccw projected
  line L119 (-5.1016, -31.6711) -> (-3.3242, -30.3798) projected
  arc A117 (-5.6005, -30.8077) -> (-5.1016, -31.6711) centre (0, -28.1477) ccw projected
  line L120 (-3.5829, -29.9094) -> (-5.6005, -30.8077) projected
  arc A118 (-3.7152, -29.6399) -> (-3.5829, -29.9094) centre (-0.061, -28.013) ccw projected
  line L121 (-5.7226, -30.5337) -> (-3.7152, -29.6399) projected
  arc A119 (-6.0311, -29.5853) -> (-5.7226, -30.5337) centre (0, -28.1477) ccw projected
  line L122 (-3.8704, -29.126) -> (-6.0311, -29.5853) projected
  arc A120 (-3.9438, -28.8349) -> (-3.8704, -29.126) centre (-0.0312, -28.0033) ccw projected
  line L123 (-6.0936, -29.2919) -> (-3.9438, -28.8349) projected
  arc A121 (-6.1982, -28.3) -> (-6.0936, -29.2919) centre (0, -28.1477) ccw projected
  arc A122 (20.4663, 10.3703) -> (20.3393, 10.1987) centre (21.202, 9.693) ccw projected
  line L124 (19.459, 11.1159) -> (20.4663, 10.3703) projected
  arc A123 (20.4246, 11.8044) -> (19.459, 11.1159) centre (21.202, 9.693) ccw projected
  line L125 (20.8013, 10.6092) -> (20.4246, 11.8044) projected
  arc A124 (21.0049, 10.6734) -> (20.8013, 10.6092) centre (21.202, 9.693) ccw projected
  line L126 (20.6282, 11.8686) -> (21.0049, 10.6734) projected
  arc A125 (21.8141, 11.8581) -> (20.6282, 11.8686) centre (21.202, 9.693) ccw projected
  line L127 (21.4164, 10.6698) -> (21.8141, 11.8581) projected
  arc A126 (21.6188, 10.602) -> (21.4164, 10.6698) centre (21.202, 9.693) ccw projected
  line L128 (22.0166, 11.7904) -> (21.6188, 10.602) projected
  arc A127 (22.9699, 11.0848) -> (22.0166, 11.7904) centre (21.202, 9.693) ccw projected
  line L129 (21.9495, 10.3572) -> (22.9699, 11.0848) projected
  arc A128 (22.0735, 10.1834) -> (21.9495, 10.3572) centre (21.202, 9.693) ccw projected
  line L130 (23.0938, 10.911) -> (22.0735, 10.1834) projected
  arc A129 (23.4503, 9.7799) -> (23.0938, 10.911) centre (21.202, 9.693) ccw projected
  line L131 (22.1972, 9.791) -> (23.4503, 9.7799) projected
  arc A130 (22.1953, 9.5775) -> (22.1972, 9.791) centre (21.202, 9.693) ccw projected
  line L132 (23.4484, 9.5664) -> (22.1953, 9.5775) projected
  arc A131 (23.072, 8.4418) -> (23.4484, 9.5664) centre (21.202, 9.693) ccw projected
  line L133 (22.0647, 9.1873) -> (23.072, 8.4418) projected
  arc A132 (21.9377, 9.0157) -> (22.0647, 9.1873) centre (21.202, 9.693) ccw projected
  line L134 (22.945, 8.2701) -> (21.9377, 9.0157) projected
  arc A133 (21.9794, 7.5816) -> (22.945, 8.2701) centre (21.202, 9.693) ccw projected
  line L135 (21.6027, 8.7768) -> (21.9794, 7.5816) projected
  arc A134 (21.3991, 8.7126) -> (21.6027, 8.7768) centre (21.202, 9.693) ccw projected
  line L136 (21.7758, 7.5174) -> (21.3991, 8.7126) projected
  arc A135 (20.5899, 7.5279) -> (21.7758, 7.5174) centre (21.202, 9.693) ccw projected
  line L137 (20.9876, 8.7162) -> (20.5899, 7.5279) projected
  arc A136 (20.7852, 8.784) -> (20.9876, 8.7162) centre (21.202, 9.693) ccw projected
  line L138 (20.3874, 7.5956) -> (20.7852, 8.784) projected
  arc A137 (19.4341, 8.3012) -> (20.3874, 7.5956) centre (21.202, 9.693) ccw projected
  line L139 (20.4545, 9.0288) -> (19.4341, 8.3012) projected
  arc A138 (20.3305, 9.2026) -> (20.4545, 9.0288) centre (21.202, 9.693) ccw projected
  line L140 (19.3102, 8.475) -> (20.3305, 9.2026) projected
  arc A139 (18.9537, 9.6061) -> (19.3102, 8.475) centre (21.202, 9.693) ccw projected
  line L141 (20.2068, 9.595) -> (18.9537, 9.6061) projected
  arc A140 (20.2087, 9.8085) -> (20.2068, 9.595) centre (21.202, 9.693) ccw projected
  line L142 (18.9556, 9.8196) -> (20.2087, 9.8085) projected
  arc A141 (19.332, 10.9442) -> (18.9556, 9.8196) centre (21.202, 9.693) ccw projected
  line L143 (20.3393, 10.1987) -> (19.332, 10.9442) projected
  line L144 (-46.4, -46.4) -> (-46.4, -41.4)
  line L145 (-46.4, 46.4) -> (-46.4, -46.4) projected
  line L146 (-46.4, -41.4) -> (-42.4, -41.4)
  line L147 (-42.4, -41.4) -> (-42.4, -46.4)
  line L148 (-46.4, -46.4) -> (46.4, -46.4) projected
  line L149 (-46.4, -46.4) -> (-42.4, -46.4)
  line L150 (-73.6925, 0) -> (63.5947, 0) construction
  line L151 (0, 77.32) -> (0, -87.2618) construction
  line L152 (46.4, 46.4) -> (46.4, -46.4)
  line L153 (46.4, -41.4) -> (42.4, -41.4)
  line L154 (42.4, -41.4) -> (42.4, -46.4)
  line L155 (46.4, -46.4) -> (-46.4, -46.4)
  line L156 (-46.4, 46.4) -> (46.4, 46.4)
  line L157 (-46.4, -46.4) -> (-46.4, 46.4)
  line L158 (-46.4, 41.4) -> (-42.4, 41.4)
  line L159 (-42.4, 41.4) -> (-42.4, 46.4)
  line L160 (42.4, 41.4) -> (42.4, 46.4)
  line L161 (46.4, 41.4) -> (42.4, 41.4)
  line L162 (46.4, -46.4) -> (46.4, 46.4)
  point P0 (0, 0)
  dimension "d61" = 5
  dimension "d62" = 4
  constraints: 34 end point, 16 symmetric about line, 4 point on line, 2 perpendicular, 1 collinear, 1 horizontal
  measures "d61" distance of L62.end L144.end
  measures "d62" distance of L144.end L146.end
extrude "Extrusion9" add sketch "Sketch7" along normal blind 3 contours L159 L158 L62 L61
mirror "Mirror3" about plane through (0, 0, -46.4) normal (-1, 0, 0) of "Extrusion9"
ref_plane "Work Plane7" through (-46.4, 0, 0) normal (0, 0, 1) x (1, 0, 0)
mirror "Mirror4" about plane through (-46.4, 0, 0) normal (0, 0, 1) of "Extrusion9", "Mirror3"
sketch "Sketch10" plane through (-46.4, 0, 46.4) normal (0, 0, 1) x (1, 0, 0)
  line L0 (0, 0) -> (92.8, 0) projected
  line L1 (92.8, 0) -> (92.8, 8) projected
  line L2 (88.8, 8) -> (92.8, 8) projected
  line L3 (88.8, 5) -> (88.8, 8) projected
  line L4 (4, 5) -> (88.8, 5) projected
  line L5 (4, 5) -> (4, 8) projected
  line L6 (4, 8) -> (0, 8) projected
  line L7 (0, 0) -> (0, 8) projected
  line L8 (4, 5) -> (0, 5) construction
  line L9 (7, 5) -> (0.5, 5) projected
  line L10 (0, 5) -> (4, 8) construction
  line L11 (0, 8) -> (4, 8) projected
  line L12 (0, 8) -> (4, 5) construction
  circle A0 centre (2, 6.5) radius 1
  point P0 (46.4, 0)
  dimension "d78" = 2
  constraints: 6 end point, 1 centre point, 1 collinear, 1 midpoint, 1 point on line
  measures "d78" diameter of A0
extrude "Extrusion12" cut sketch "Sketch10" against normal up to surface (5 mm away) contours A0
mirror "Mirror8" about plane through (0, 0, -46.4) normal (-1, 0, 0) of "Extrusion12"
mirror "Mirror9" about plane through (-46.4, 0, 0) normal (0, 0, 1) of "Extrusion12", "Mirror8"